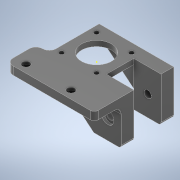
# Autodesk Inventor part: NEMA14 support
Saved by Autodesk Inventor 2022 (Build 260153000, 153)
## iProperties
Created: 2022-03-06
Part Number: NEMA14 support
Material: Genérico
Document SubType Name: Modeling
Designer: JK
Density: 1 g/cm^3
Appearance: Suave - Negro
Author: JK
Autodesk Inventor part; units mm, degrees
ref_plane "YZ Plane" through (0, 0, 0) normal (1, 0, 0) x (0, 1, 0)
ref_plane "XZ Plane" through (0, 0, 0) normal (0, 1, 0) x (-1, 0, 0)
ref_plane "XY Plane" through (0, 0, 0) normal (0, 0, 1) x (1, 0, 0)
sketch "Boceto1" plane through (0, 0, 0) normal (0, 1, 0) x (-1, 0, 0)
  line L0 (-17.55, 17.55) -> (17.55, 17.55)
  line L1 (17.55, 17.55) -> (17.55, -17.55)
  line L2 (17.55, -17.55) -> (-17.55, -17.55)
  line L3 (-17.55, -17.55) -> (-17.55, 17.55)
  line L4 (-17.55, 17.55) -> (17.55, -17.55) construction
  line L5 (17.55, 17.55) -> (-17.55, -17.55) construction
  circle A0 centre (0, 0) radius 11.2
  point P0 (0, 0)
  dimension "d0" = 35.1
  dimension "d1" = 35.1
  dimension "d2" = 22.4
  constraints: 12 end point, 2 midpoint, 2 parallel, 1 centre point, 1 coincident, 1 horizontal, 1 perpendicular
  measures "d0" distance of L0.end L1.end
  measures "d1" distance of L1.end L2.end
  measures "d2" diameter of A0
extrude "Extrusión1" add sketch "Boceto1" along normal blind 4
sketch "Boceto2" plane through (0, 4, 0) normal (0, 1, 0) x (1, 0, 0)
  circle A0 centre (-13, -13) radius 1.7
  line L0 (13, -13) -> (-13, -13)
  line L1 (-13, -13) -> (-13, 13)
  line L2 (-13, 13) -> (13, 13)
  line L3 (13, 13) -> (13, -13)
  line L4 (13, -13) -> (-13, 13) construction
  line L5 (-13, -13) -> (13, 13) construction
  point P0 (0, 0)
  dimension "d5" = 26
  dimension "d6" = 26
  dimension "d7" = 3.4
  constraints: 12 end point, 2 midpoint, 2 parallel, 1 centre point, 1 coincident, 1 horizontal, 1 perpendicular
  measures "d5" distance of L1.end L2.end
  measures "d6" distance of L0.end L1.end
  measures "d7" diameter of A0
extrude "Extrusión2" cut sketch "Boceto2" against normal through all contours L0 L1 A0 | A0 L1 L0
pattern_circular "Patrón circular1" count 4 over 360 about axis through (0, 0, 0) along (0, 1, 0) of "Extrusión2"
sketch "Boceto13" plane through (0, 4, 0) normal (0, 1, 0) x (1, 0, 0)
  line L0 (-17.55, -17.55) -> (17.55, -17.55) projected
  line L1 (17.55, -17.55) -> (37.85, -17.55)
  line L2 (37.85, -17.55) -> (37.85, 17.55)
  line L3 (37.85, 17.55) -> (17.55, 17.55)
  line L4 (17.55, 17.55) -> (17.55, -17.55)
  line L5 (17.55, 17.55) -> (-17.55, 17.55) projected
  line L6 (41.5, -10.15) -> (21.2, -10.15)
  line L7 (21.2, -10.15) -> (21.2, 10.15)
  line L8 (21.2, 10.15) -> (41.5, 10.15)
  line L9 (41.5, 10.15) -> (41.5, -10.15)
  line L10 (41.5, -10.15) -> (21.2, 10.15) construction
  line L11 (21.2, -10.15) -> (41.5, 10.15) construction
  circle A0 centre (27.85, 0) radius 2.7
  point P0 (0, 0)
  point P1 (31.35, 0)
  dimension "d43" = 20.3
  dimension "d44" = 20.3
  dimension "d45" = 20.3
  dimension "d61" = 5.4
  dimension "d62" = 10
  constraints: 20 end point, 4 parallel, 2 horizontal, 2 midpoint, 2 perpendicular, 1 centre point, 1 collinear
  measures "d43" distance of L2.end L3.end
  measures "d44" distance of L7.end L8.end
  measures "d45" distance of L6.end L7.end
  measures "d61" diameter of A0
  measures "d62" distance from line of L2 A0.centre
extrude "Extrusión8" add sketch "Boceto13" against normal blind 33 contours L4 L3 L2 L8 L7 L6 L1 | L6 L7 L8 L2
sketch "Boceto14" plane through (0, -29, 0) normal (0, -1, 0) x (1, 0, 0)
  line L0 (17.55, 17.55) -> (17.55, -17.55) projected
  line L1 (37.85, -10.15) -> (17.55, -10.15)
  line L2 (17.55, -10.15) -> (17.55, 10.15)
  line L3 (17.55, 10.15) -> (37.85, 10.15)
  line L4 (37.85, 10.15) -> (37.85, -10.15)
  line L5 (37.85, -10.15) -> (17.55, 10.15) construction
  line L6 (17.55, -10.15) -> (37.85, 10.15) construction
  line L7 (37.85, -17.55) -> (37.85, 17.55) projected
  circle A0 centre (27.85, 0) radius 2.7 projected
  point P0 (0, 0)
  point P1 (27.7, 0)
  point P2 (17.55, -10.15)
  point P3 (27.7, 0)
  dimension "d49" = 20.3
  constraints: 12 end point, 3 midpoint, 2 parallel, 1 collinear, 1 horizontal, 1 horizontal alignment, 1 perpendicular, 1 point on line
  measures "d49" distance between parallel lines of L3 L1
extrude "Extrusión9" cut sketch "Boceto14" against normal up to surface (29 mm away) contours L3 L4 L1 L0 | A0
sketch "Boceto15" plane through (-17.55, 0, -17.55) normal (0, 0, -1) x (-1, 0, 0)
  line L0 (-35.1, 0) -> (0, 0) projected
  line L1 (0, 0) -> (0, 4) projected
  line L2 (-55.4, 4) -> (0, 4) projected
  line L3 (-55.4, 4) -> (-55.4, -29) projected
  line L4 (-35.1, -29) -> (-55.4, -29) projected
  line L5 (-35.1, 0) -> (-35.1, -29) projected
  line L6 (0, 0) -> (0, 4) projected
  line L7 (-35.1, -29) -> (-55.4, -29) projected
  line L8 (0, 0) -> (-35.1, -29)
  point P0 (-17.55, 0)
  constraints: 2 end point
extrude "Extrusión10" add sketch "Boceto15" along normal blind 2
mirror "Simetría1" about plane through (0, 0, 0) normal (0, 0, 1) of "Extrusión10"
sketch "Boceto16" plane through (-17.55, 0, -19.55) normal (0, 0, -1) x (-1, 0, 0)
  circle A0 centre (-45.4, -14) radius 2.7
  line L0 (-55.4, 4) -> (-55.4, -29) projected
  line L1 (-55.4, -29) -> (-35.1, -29) projected
  point P0 (-17.55, 0)
  dimension "d54" = 10
  dimension "d55" = 5.4
  dimension "d57" = 15
  constraints: 1 centre point
  measures "d54" distance from line of L0 A0.centre
  measures "d55" diameter of A0
  measures "d57" distance from line of L1 A0.centre
extrude "Extrusión11" cut sketch "Boceto16" against normal through all
fillet "Empalme1" radius 2 1 edges at (37.85, -29, -14.85)
sketch "Boceto17" plane through (-17.55, 0, -19.55) normal (0, 0, -1) x (-1, 0, 0)
  circle A0 centre (-45.4, -14) radius 2.7 projected
  circle A1 centre (-45.4, -14) radius 4.65
  point P0 (-17.55, 0)
  dimension "d63" = 9.3
  constraints: 1 centre point, 1 coincident
  measures "d63" diameter of A1
extrude "Extrusión12" cut sketch "Boceto17" against normal blind 2 contours A0 | A1
sketch "Boceto18" plane through (0, 4, 0) normal (0, 1, 0) x (1, 0, 0)
  circle A0 centre (27.85, 0) radius 2.7 projected
  circle A1 centre (27.85, 0) radius 4.6
  point P0 (0, 0)
  dimension "d66" = 9.2
  constraints: 1 centre point, 1 coincident
  measures "d66" diameter of A1
extrude "Extrusión13" cut sketch "Boceto18" against normal blind 2 contours A0 | A1
mirror "Simetría2" about plane through (0, 0, 0) normal (0, 0, 1) of "Extrusión12"
sketch "Boceto19" plane through (0, 4, 0) normal (0, 1, 0) x (1, 0, 0)
  line L0 (17.55, -17.55) -> (-17.55, -17.55) projected
  line L1 (-17.55, 17.55) -> (-17.55, -17.55) projected
  line L2 (-17.55, -17.55) -> (37.85, -17.55)
  line L3 (37.85, -17.55) -> (37.85, -39.55)
  line L4 (37.85, -39.55) -> (-17.55, -39.55)
  line L5 (-17.55, -39.55) -> (-17.55, -17.55)
  line L6 (-17.55, -19.55) -> (37.85, -19.55) projected
  line L7 (37.85, -19.55) -> (37.85, 19.55) projected
  line L8 (-17.55, -17.55) -> (-17.55, -19.55) projected
  line L9 (-17.55, -17.55) -> (-27.55, -17.55)
  line L10 (-27.55, -17.55) -> (-27.55, -39.55)
  line L11 (-27.55, -39.55) -> (-17.55, -39.55)
  line L12 (-17.55, -39.55) -> (-17.55, -17.55)
  point P0 (0, 0)
  dimension "d69" = 20
  dimension "d86" = 10
  constraints: 16 end point, 4 parallel, 2 collinear, 2 horizontal, 2 perpendicular
  measures "d69" distance between parallel lines of L6 L4
  measures "d86" distance between parallel lines of L10 L5
extrude "Extrusión14" add sketch "Boceto19" against normal blind 6
sketch "Boceto20" plane through (0, -2, 0) normal (0, -1, 0) x (1, 0, 0)
  circle A0 centre (-18.875, 33.55) radius 2.7
  circle A1 centre (14.55, 33.55) radius 2.7
  line L0 (37.85, 19.55) -> (37.85, 39.55) projected
  line L1 (-27.55, 39.55) -> (-27.55, 17.55) projected
  line L2 (37.85, 39.55) -> (-27.55, 39.55) projected
  point P0 (0, 0)
  dimension "d72" = 5.4
  dimension "d74" = 23.3
  dimension "d87" = 8.675
  dimension "d88" = 6
  constraints: 2 centre point, 1 equal radius, 1 horizontal alignment
  measures "d72" diameter of A0
  measures "d74" distance from line of A1.centre L0
  measures "d87" distance from line of L1 A0.centre
  measures "d88" distance from line of L2 A0.centre
extrude "Extrusión15" cut sketch "Boceto20" against normal through all
sketch "Boceto21" plane through (0, -2, 0) normal (0, -1, 0) x (1, 0, 0)
  circle A0 centre (-18.875, 33.55) radius 2.7 projected
  circle A1 centre (-18.875, 33.55) radius 4.05
  circle A2 centre (14.55, 33.55) radius 2.7 projected
  circle A3 centre (14.55, 33.55) radius 4.05
  line L0 (14.55, 38.2265) -> (18.6, 35.8883)
  line L1 (18.6, 35.8883) -> (18.6, 31.2117)
  line L2 (18.6, 31.2117) -> (14.55, 28.8735)
  line L3 (14.55, 28.8735) -> (10.5, 31.2117)
  line L4 (10.5, 31.2117) -> (10.5, 35.8883)
  line L5 (10.5, 35.8883) -> (14.55, 38.2265)
  line L6 (-18.875, 38.2265) -> (-14.825, 35.8883)
  line L7 (-14.825, 35.8883) -> (-14.825, 31.2117)
  line L8 (-14.825, 31.2117) -> (-18.875, 28.8735)
  line L9 (-18.875, 28.8735) -> (-22.925, 31.2117)
  line L10 (-22.925, 31.2117) -> (-22.925, 35.8883)
  line L11 (-22.925, 35.8883) -> (-18.875, 38.2265)
  point P0 (0, 0)
  dimension "d79" = 8.1
  constraints: 24 end point, 4 coincident, 2 centre point, 2 tangent, 2 vertical, 1 equal radius, 26 other
  measures "d79" diameter of A3
extrude "Extrusión16" cut sketch "Boceto21" against normal blind 4 contours A0 | A1 | L7 L8 A1 | A1 L6 L7 | A1 L11 L6 | L8 L9 A1 | A1 L10 L11 | L9 L10 A1 | A2 | A3 | L1 L2 A3 | A3 L0 L1 | A3 L5 L0 | L2 L3 A3 | A3 L4 L5 | L3 L4 A3
fillet "Empalme2" radius 3 1 edges at (37.85, 1, 39.55)
fillet "Empalme3" radius 5 1 edges at (11.3603, -2, 19.55)
sketch "Boceto22" plane through (0, 4, 0) normal (0, 1, 0) x (1, 0, 0)
  line L0 (37.85, -10.15) -> (37.85, 10.15) projected
  line L1 (35.85, 10.15) -> (17.55, 10.15) projected
  line L2 (37.85, -10.15) -> (17.55, -10.15)
  line L3 (17.55, -10.15) -> (17.55, 10.15)
  line L4 (17.55, 10.15) -> (37.85, 10.15)
  line L5 (37.85, 10.15) -> (37.85, -10.15)
  line L6 (17.55, 10.15) -> (17.55, 17.55) projected
  point P0 (0, 0)
  constraints: 8 end point, 2 parallel, 1 collinear, 1 horizontal, 1 perpendicular, 1 point on line
extrude "Extrusión17" cut sketch "Boceto22" against normal through all
fillet "Empalme4" radius 5 3 edges at (-27.55, 1, 39.55) (-27.55, 1, 17.55) (-17.55, 2, 17.55)
sketch "Boceto24" plane through (0, -2, 0) normal (0, -1, 0) x (1, 0, 0)
  point P0 (0, 0)
  constraints: 1 centre point
sketch "Boceto7" plane through (17.55, 0, -17.55) normal (0, 0, -1) x (-1, 0, 0)
  line L0 (35.1, 0) -> (35.1, 4) projected
  line L1 (35.1, 4) -> (-20.3, 4)
  line L2 (-20.3, 4) -> (-20.3, -26)
  line L3 (-20.3, -26) -> (35.1, -26)
  line L4 (35.1, -26) -> (35.1, 4)
  line L5 (0, 0) -> (0, 4) projected
  point P0 (17.55, 0)
  point P1 (35.6, 0)
  dimension "d23" = 20.3
  dimension "d24" = 30
  constraints: 8 end point, 2 parallel, 1 horizontal, 1 perpendicular
  measures "d23" distance between parallel lines of L2 L5
  measures "d24" distance between parallel lines of L1 L3
sketch "Boceto8" plane through (0, 3, 0) normal (0, 1, 0) x (1, 0, 0)
  line L0 (17.8, 17.8) -> (-17.8, 17.8) projected
  line L1 (17.8, -17.8) -> (16.8, -17.8)
  line L2 (16.8, -17.8) -> (16.8, 17.8)
  line L3 (16.8, 17.8) -> (17.8, 17.8)
  line L4 (17.8, 17.8) -> (17.8, -17.8)
  point P0 (0, 0)
  dimension "d27" = 1
  constraints: 8 end point, 2 parallel, 1 horizontal, 1 perpendicular, 1 point on line
  measures "d27" distance between parallel lines of L2 L4
sketch "Boceto9" plane through (17.8, 0, -21.8) normal (0, 0, -1) x (-1, 0, 0)
  circle A0 centre (-10.3, -4.5) radius 2.7
  circle A1 centre (-10.3, -19.5) radius 2.7
  line L0 (-20.3, 3) -> (-20.3, -27) projected
  line L1 (35.6, 3) -> (-20.3, 3) projected
  line L2 (-20.3, -27) -> (35.6, -27) projected
  point P0 (17.8, 0)
  dimension "d30" = 5.4
  dimension "d31" = 10
  dimension "d32" = 7.5
  dimension "d33" = 7.5
  dimension "d41" = 80
  dimension "d42" = 20.3
  constraints: 12 end point, 2 midpoint, 2 parallel, 1 horizontal, 1 perpendicular
  measures "d41" distance of L1.end L2.end
  measures "d42" distance of L0.end L1.end
sketch "Boceto10" plane through (17.8, 0, -17.8) normal (0, 0, 1) x (1, 0, 0)
  line L0 (20.3, 3) -> (20.3, -27) projected
  line L1 (-1, 3) -> (20.3, 3) projected
  line L2 (20.3, -27) -> (0.3, -27)
  line L3 (0.3, -27) -> (0.3, 3)
  line L4 (0.3, 3) -> (20.3, 3)
  line L5 (20.3, 3) -> (20.3, -27)
  circle A0 centre (10.3, -4.5) radius 2.7 projected
  circle A1 centre (10.3, -19.5) radius 2.7 projected
  line L6 (-1, 0) -> (-35.6, 0) projected
  line L7 (-35.6, -27) -> (-35.6, 0) projected
  line L8 (20.3, -27) -> (-35.6, -27) projected
  line L9 (20.3, 3) -> (20.3, -27) projected
  line L10 (-1, 3) -> (20.3, 3) projected
  line L11 (-1, 3) -> (-1, 0) projected
  point P0 (-17.8, 0)
  dimension "d36" = 20
  constraints: 8 end point, 2 parallel, 1 horizontal, 1 perpendicular, 1 point on line
  measures "d36" distance of L3.end L4.end
sketch "Boceto3" plane through (-17.55, 0, 17.55) normal (0, 0, 1) x (1, 0, 0)
  line L0 (0, 0) -> (0, 4) projected
  line L1 (0, 4) -> (55.4, 4)
  line L2 (55.4, 4) -> (55.4, -30)
  line L3 (55.4, -30) -> (0, -30)
  line L4 (0, -30) -> (0, 4)
  line L5 (35.1, 0) -> (35.1, 4) projected
  line L6 (0, 0) -> (35.1, 0) projected
  point P0 (17.55, 0)
  dimension "d13" = 20.3
  dimension "d14" = 30
  dimension "d17" = 5.4
  dimension "d18" = 10
  dimension "d19" = 7.5
  dimension "d20" = 7.5
  dimension "d21" = 20.3
  dimension "d22" = 20.3
  constraints: 8 end point, 2 parallel, 1 horizontal, 1 perpendicular
  measures "d21" distance of L1.end L2.end
  measures "d22" distance of L0.end L1.end
